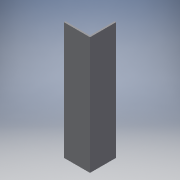
# Autodesk Inventor part: OTHER bracket for pickup
Saved by Autodesk Inventor 2017 (Build 210142000, 142)
## iProperties
Created: 2016-12-03
Part Number: OTHER bracket for pickup
Material: Generic
Document SubType Name: Modeling
Designer: Aditya
Density: 1 g/cm^3
Appearance: Default
Author: Aditya
Autodesk Inventor part; units mm, degrees
ref_plane "YZ Plane" through (0, 0, 0) normal (1, 0, 0) x (0, 1, 0)
ref_plane "XZ Plane" through (0, 0, 0) normal (0, 1, 0) x (-1, 0, 0)
ref_plane "XY Plane" through (0, 0, 0) normal (0, 0, 1) x (1, 0, 0)
sketch "Sketch1" plane through (0, 0, 0) normal (0, 1, 0) x (-1, 0, 0)
  line L0 (0, 0) -> (0, -25.4)
  line L1 (0, -25.4) -> (1.5875, -25.4)
  line L2 (0, 0) -> (25.4, 0)
  line L3 (25.4, 0) -> (25.4, -1.5875)
  line L4 (25.4, -1.5875) -> (1.5875, -1.5875)
  line L5 (1.5875, -1.5875) -> (1.5875, -25.4)
  dimension "d0" = 25.4
  dimension "d1" = 1.5875
  dimension "d4" = 25.4
  dimension "d5" = 1.5875
  constraints: 12 end point, 2 perpendicular, 2 vertical, 1 horizontal
  measures "d0" distance of L0.start L0.end
  measures "d1" distance of L0.end L1.end
  measures "d4" distance of L0.start L2.end
  measures "d5" distance of L2.end L3.end
extrude "Extrusion1" add sketch "Sketch1" along normal blind 114.3
body "Solid1"
